Autodesk Inventor part; units mm, degrees
(part 2 of 2)
  line L285 (-19.9642, -36.6708) -> (-19.322, -36.6708)
  line L286 (-19.322, -36.6708) -> (-19.322, -35.0579)
  line L287 (-19.322, -35.0579) -> (-19.9642, -35.0579)
  line L288 (-19.9642, -35.0579) -> (-19.9642, -34.5614)
  spline S239 degree 2 poles (-19.9642, -34.5614) (-19.8234, -34.5614) (-19.5443, -34.5244) (-19.4603, -34.4848) knots 0 0 0 1 2 2 2
  spline S240 degree 2 poles (-19.4603, -34.4848) (-19.3639, -34.4354) (-19.2553, -34.27) (-19.2454, -34.1465) knots 0 0 0 1 2 2 2
  line L289 (-19.2454, -34.1465) -> (-18.5785, -34.1465)
  line L290 (-18.5785, -34.1465) -> (-18.5785, -36.6708)
  line L291 (-18.5785, -36.6708) -> (-17.9511, -36.6708)
  line L292 (-17.9511, -36.6708) -> (-17.9511, -37.2019)
  spline S241 degree 2 poles (-15.1624, -36.1645) (-15.1624, -36.6461) (-15.7725, -37.2661) (-16.3061, -37.2661) knots 0 0 0 1 2 2 2
  spline S242 degree 2 poles (-16.3061, -37.2661) (-16.5728, -37.2661) (-16.9903, -37.1129) (-17.136, -36.9623) knots 0 0 0 1 2 2 2
  spline S243 degree 2 poles (-17.136, -36.9623) (-17.3089, -36.7869) (-17.4941, -36.2312) (-17.4941, -35.8434) knots 0 0 0 1 2 2 2
  spline S244 degree 2 poles (-17.4941, -35.8434) (-17.4941, -35.4432) (-17.3212, -34.8208) (-17.1261, -34.5812) knots 0 0 0 1 2 2 2
  spline S245 degree 2 poles (-17.1261, -34.5812) (-16.9409, -34.3539) (-16.3382, -34.0971) (-15.9257, -34.0971) knots 0 0 0 1 2 2 2
  spline S246 degree 2 poles (-15.9257, -34.0971) (-15.775, -34.0971) (-15.4737, -34.1366) (-15.4193, -34.1489) knots 0 0 0 1 2 2 2
  line L293 (-15.4193, -34.1489) -> (-15.4193, -34.7467)
  line L294 (-15.4193, -34.7467) -> (-15.4737, -34.7467)
  spline S247 degree 2 poles (-15.4737, -34.7467) (-15.528, -34.7195) (-15.775, -34.6528) (-15.9331, -34.6528) knots 0 0 0 1 2 2 2
  spline S248 degree 2 poles (-15.9331, -34.6528) (-16.2912, -34.6528) (-16.6815, -35.0307) (-16.7284, -35.3815) knots 0 0 0 1 2 2 2
  spline S249 degree 2 poles (-16.7284, -35.3815) (-16.5778, -35.2851) (-16.269, -35.1715) (-16.0739, -35.1715) knots 0 0 0 1 2 2 2
  spline S250 degree 2 poles (-16.0739, -35.1715) (-15.9084, -35.1715) (-15.6194, -35.2604) (-15.5083, -35.3444) knots 0 0 0 1 2 2 2
  spline S251 degree 2 poles (-15.5083, -35.3444) (-15.3502, -35.4654) (-15.1624, -35.8582) (-15.1624, -36.1645) knots 0 0 0 1 2 2 2
  spline S252 degree 2 poles (-16.0541, -36.6239) (-15.9948, -36.5498) (-15.9306, -36.3769) (-15.9306, -36.2015) knots 0 0 0 1 2 2 2
  spline S253 degree 2 poles (-15.9306, -36.2015) (-15.9306, -36.0533) (-16.0047, -35.8606) (-16.0714, -35.8038) knots 0 0 0 1 2 2 2
  spline S254 degree 2 poles (-16.0714, -35.8038) (-16.1406, -35.7446) (-16.311, -35.7026) (-16.4073, -35.7026) knots 0 0 0 1 2 2 2
  spline S255 degree 2 poles (-16.4073, -35.7026) (-16.4888, -35.7026) (-16.6568, -35.7446) (-16.7309, -35.7742) knots 0 0 0 1 2 2 2
  spline S256 degree 2 poles (-16.7309, -35.7742) (-16.7309, -35.794) (-16.7359, -35.8878) (-16.7359, -35.9594) knots 0 0 0 1 2 2 2
  spline S257 degree 2 poles (-16.7359, -35.9594) (-16.7359, -36.2237) (-16.6445, -36.5424) (-16.5728, -36.6239) knots 0 0 0 1 2 2 2
  spline S258 degree 2 poles (-16.5728, -36.6239) (-16.521, -36.6906) (-16.3826, -36.7474) (-16.3085, -36.7474) knots 0 0 0 1 2 2 2
  spline S259 degree 2 poles (-16.3085, -36.7474) (-16.2468, -36.7474) (-16.1035, -36.6856) (-16.0541, -36.6239) knots 0 0 0 1 2 2 2
  line L295 (-12.8061, -37.2019) -> (-13.5224, -37.2019)
  line L296 (-13.5224, -37.2019) -> (-13.5224, -34.9023)
  line L297 (-13.5224, -34.9023) -> (-12.8061, -34.9023)
  line L298 (-12.8061, -34.9023) -> (-12.8061, -37.2019)
  line L299 (-12.7838, -34.5738) -> (-13.5421, -34.5738)
  line L300 (-13.5421, -34.5738) -> (-13.5421, -34.0155)
  line L301 (-13.5421, -34.0155) -> (-12.7838, -34.0155)
  line L302 (-12.7838, -34.0155) -> (-12.7838, -34.5738)
  line L303 (-10.1063, -37.2019) -> (-10.8276, -37.2019)
  line L304 (-10.8276, -37.2019) -> (-10.8276, -36.0632)
  spline S260 degree 2 poles (-10.8276, -36.0632) (-10.8276, -35.9224) (-10.8498, -35.6458) (-10.8794, -35.5815) knots 0 0 0 1 2 2 2
  spline S261 degree 2 poles (-10.8794, -35.5815) (-10.9165, -35.5025) (-11.0548, -35.4358) (-11.1734, -35.4358) knots 0 0 0 1 2 2 2
  spline S262 degree 2 poles (-11.1734, -35.4358) (-11.2598, -35.4358) (-11.4401, -35.5025) (-11.5414, -35.5741) knots 0 0 0 1 2 2 2
  line L305 (-11.5414, -35.5741) -> (-11.5414, -37.2019)
  line L306 (-11.5414, -37.2019) -> (-12.2577, -37.2019)
  line L307 (-12.2577, -37.2019) -> (-12.2577, -34.9023)
  line L308 (-12.2577, -34.9023) -> (-11.5414, -34.9023)
  line L309 (-11.5414, -34.9023) -> (-11.5414, -35.1567)
  spline S263 degree 2 poles (-11.5414, -35.1567) (-11.366, -35.0085) (-11.0326, -34.8405) (-10.83, -34.8405) knots 0 0 0 1 2 2 2
  spline S264 degree 2 poles (-10.83, -34.8405) (-10.4793, -34.8405) (-10.1063, -35.2851) (-10.1063, -35.705) knots 0 0 0 1 2 2 2
  line L310 (-10.1063, -35.705) -> (-10.1063, -37.2019)
  spline S265 degree 2 poles (-8.4489, -37.2636) (-8.733, -37.2636) (-9.2048, -37.1204) (-9.3801, -36.9722) knots 0 0 0 1 2 2 2
  spline S266 degree 2 poles (-9.3801, -36.9722) (-9.5506, -36.8215) (-9.7432, -36.3695) (-9.7432, -36.0632) knots 0 0 0 1 2 2 2
  spline S267 degree 2 poles (-9.7432, -36.0632) (-9.7432, -35.7322) (-9.5358, -35.2703) (-9.3554, -35.1221) knots 0 0 0 1 2 2 2
  spline S268 degree 2 poles (-9.3554, -35.1221) (-9.185, -34.9789) (-8.7206, -34.8405) (-8.4687, -34.8405) knots 0 0 0 1 2 2 2
  spline S269 degree 2 poles (-8.4687, -34.8405) (-8.2785, -34.8405) (-7.8981, -34.9295) (-7.7055, -35.0258) knots 0 0 0 1 2 2 2
  line L311 (-7.7055, -35.0258) -> (-7.7055, -35.6383)
  line L312 (-7.7055, -35.6383) -> (-7.7969, -35.6383)
  spline S270 degree 2 poles (-7.7969, -35.6383) (-7.8413, -35.5964) (-7.9648, -35.4976) (-8.0389, -35.458) knots 0 0 0 1 2 2 2
  spline S271 degree 2 poles (-8.0389, -35.458) (-8.118, -35.4136) (-8.3131, -35.3543) (-8.4341, -35.3543) knots 0 0 0 1 2 2 2
  spline S272 degree 2 poles (-8.4341, -35.3543) (-8.7083, -35.3543) (-9.0096, -35.7371) (-9.0096, -36.0632) knots 0 0 0 1 2 2 2
  spline S273 degree 2 poles (-9.0096, -36.0632) (-9.0096, -36.409) (-8.6885, -36.7499) (-8.4218, -36.7499) knots 0 0 0 1 2 2 2
  spline S274 degree 2 poles (-8.4218, -36.7499) (-8.2859, -36.7499) (-8.0834, -36.6881) (-8.0093, -36.6436) knots 0 0 0 1 2 2 2
  spline S275 degree 2 poles (-8.0093, -36.6436) (-7.9377, -36.6017) (-7.8339, -36.5078) (-7.7969, -36.4707) knots 0 0 0 1 2 2 2
  line L313 (-7.7969, -36.4707) -> (-7.7055, -36.4707)
  line L314 (-7.7055, -36.4707) -> (-7.7055, -37.0858)
  spline S276 degree 2 poles (-7.7055, -37.0858) (-7.7672, -37.1129) (-7.9278, -37.1821) (-8.0118, -37.2043) knots 0 0 0 1 2 2 2
  spline S277 degree 2 poles (-8.0118, -37.2043) (-8.1155, -37.234) (-8.2983, -37.2636) (-8.4489, -37.2636) knots 0 0 0 1 2 2 2
  line L315 (-5.2132, -37.2019) -> (-5.9345, -37.2019)
  line L316 (-5.9345, -37.2019) -> (-5.9345, -36.0632)
  spline S278 degree 2 poles (-5.9345, -36.0632) (-5.9345, -35.9224) (-5.9567, -35.6458) (-5.9863, -35.5815) knots 0 0 0 1 2 2 2
  spline S279 degree 2 poles (-5.9863, -35.5815) (-6.0234, -35.5025) (-6.1617, -35.4358) (-6.2803, -35.4358) knots 0 0 0 1 2 2 2
  spline S280 degree 2 poles (-6.2803, -35.4358) (-6.3667, -35.4358) (-6.547, -35.5025) (-6.6483, -35.5741) knots 0 0 0 1 2 2 2
  line L317 (-6.6483, -35.5741) -> (-6.6483, -37.2019)
  line L318 (-6.6483, -37.2019) -> (-7.3646, -37.2019)
  line L319 (-7.3646, -37.2019) -> (-7.3646, -34.018)
  line L320 (-7.3646, -34.018) -> (-6.6483, -34.018)
  line L321 (-6.6483, -34.018) -> (-6.6483, -35.1567)
  spline S281 degree 2 poles (-6.6483, -35.1567) (-6.4729, -35.0085) (-6.1395, -34.8405) (-5.9369, -34.8405) knots 0 0 0 1 2 2 2
  spline S282 degree 2 poles (-5.9369, -34.8405) (-5.5862, -34.8405) (-5.2132, -35.2851) (-5.2132, -35.705) knots 0 0 0 1 2 2 2
  line L322 (-5.2132, -35.705) -> (-5.2132, -37.2019)
  line L323 (7.0212, -34.759) -> (5.7195, -37.2019)
  line L324 (5.7195, -37.2019) -> (4.8698, -37.2019)
  line L325 (4.8698, -37.2019) -> (6.2307, -34.7294)
  line L326 (6.2307, -34.7294) -> (4.7784, -34.7294)
  line L327 (4.7784, -34.7294) -> (4.7784, -34.1539)
  line L328 (4.7784, -34.1539) -> (7.0212, -34.1539)
  line L329 (7.0212, -34.1539) -> (7.0212, -34.759)
  line L330 (9.2516, -34.018) -> (8.0388, -37.8638)
  line L331 (8.0388, -37.8638) -> (7.4509, -37.8638)
  line L332 (7.4509, -37.8638) -> (8.6612, -34.018)
  line L333 (8.6612, -34.018) -> (9.2516, -34.018)
  spline S283 degree 2 poles (12.1588, -36.1645) (12.1588, -36.6461) (11.5487, -37.2661) (11.0152, -37.2661) knots 0 0 0 1 2 2 2
  spline S284 degree 2 poles (11.0152, -37.2661) (10.7484, -37.2661) (10.331, -37.1129) (10.1852, -36.9623) knots 0 0 0 1 2 2 2
  spline S285 degree 2 poles (10.1852, -36.9623) (10.0123, -36.7869) (9.8271, -36.2312) (9.8271, -35.8434) knots 0 0 0 1 2 2 2
  spline S286 degree 2 poles (9.8271, -35.8434) (9.8271, -35.4432) (10, -34.8208) (10.1951, -34.5812) knots 0 0 0 1 2 2 2
  spline S287 degree 2 poles (10.1951, -34.5812) (10.3804, -34.3539) (10.9831, -34.0971) (11.3956, -34.0971) knots 0 0 0 1 2 2 2
  spline S288 degree 2 poles (11.3956, -34.0971) (11.5462, -34.0971) (11.8476, -34.1366) (11.9019, -34.1489) knots 0 0 0 1 2 2 2
  line L334 (11.9019, -34.1489) -> (11.9019, -34.7467)
  line L335 (11.9019, -34.7467) -> (11.8476, -34.7467)
  spline S289 degree 2 poles (11.8476, -34.7467) (11.7932, -34.7195) (11.5462, -34.6528) (11.3881, -34.6528) knots 0 0 0 1 2 2 2
  spline S290 degree 2 poles (11.3881, -34.6528) (11.03, -34.6528) (10.6397, -35.0307) (10.5928, -35.3815) knots 0 0 0 1 2 2 2
  spline S291 degree 2 poles (10.5928, -35.3815) (10.7435, -35.2851) (11.0522, -35.1715) (11.2474, -35.1715) knots 0 0 0 1 2 2 2
  spline S292 degree 2 poles (11.2474, -35.1715) (11.4128, -35.1715) (11.7018, -35.2604) (11.813, -35.3444) knots 0 0 0 1 2 2 2
  spline S293 degree 2 poles (11.813, -35.3444) (11.9711, -35.4654) (12.1588, -35.8582) (12.1588, -36.1645) knots 0 0 0 1 2 2 2
  spline S294 degree 2 poles (11.2671, -36.6239) (11.3264, -36.5498) (11.3906, -36.3769) (11.3906, -36.2015) knots 0 0 0 1 2 2 2
  spline S295 degree 2 poles (11.3906, -36.2015) (11.3906, -36.0533) (11.3165, -35.8606) (11.2498, -35.8038) knots 0 0 0 1 2 2 2
  spline S296 degree 2 poles (11.2498, -35.8038) (11.1807, -35.7446) (11.0102, -35.7026) (10.9139, -35.7026) knots 0 0 0 1 2 2 2
  spline S297 degree 2 poles (10.9139, -35.7026) (10.8324, -35.7026) (10.6644, -35.7446) (10.5903, -35.7742) knots 0 0 0 1 2 2 2
  spline S298 degree 2 poles (10.5903, -35.7742) (10.5903, -35.794) (10.5854, -35.8878) (10.5854, -35.9594) knots 0 0 0 1 2 2 2
  spline S299 degree 2 poles (10.5854, -35.9594) (10.5854, -36.2237) (10.6768, -36.5424) (10.7484, -36.6239) knots 0 0 0 1 2 2 2
  spline S300 degree 2 poles (10.7484, -36.6239) (10.8003, -36.6906) (10.9386, -36.7474) (11.0127, -36.7474) knots 0 0 0 1 2 2 2
  spline S301 degree 2 poles (11.0127, -36.7474) (11.0744, -36.7474) (11.2177, -36.6856) (11.2671, -36.6239) knots 0 0 0 1 2 2 2
  line L336 (14.5152, -37.2019) -> (13.7989, -37.2019)
  line L337 (13.7989, -37.2019) -> (13.7989, -34.9023)
  line L338 (13.7989, -34.9023) -> (14.5152, -34.9023)
  line L339 (14.5152, -34.9023) -> (14.5152, -37.2019)
  line L340 (14.5374, -34.5738) -> (13.7791, -34.5738)
  line L341 (13.7791, -34.5738) -> (13.7791, -34.0155)
  line L342 (13.7791, -34.0155) -> (14.5374, -34.0155)
  line L343 (14.5374, -34.0155) -> (14.5374, -34.5738)
  line L344 (17.2149, -37.2019) -> (16.4937, -37.2019)
  line L345 (16.4937, -37.2019) -> (16.4937, -36.0632)
  spline S302 degree 2 poles (16.4937, -36.0632) (16.4937, -35.9224) (16.4714, -35.6458) (16.4418, -35.5815) knots 0 0 0 1 2 2 2
  spline S303 degree 2 poles (16.4418, -35.5815) (16.4047, -35.5025) (16.2664, -35.4358) (16.1479, -35.4358) knots 0 0 0 1 2 2 2
  spline S304 degree 2 poles (16.1479, -35.4358) (16.0614, -35.4358) (15.8811, -35.5025) (15.7798, -35.5741) knots 0 0 0 1 2 2 2
  line L346 (15.7798, -35.5741) -> (15.7798, -37.2019)
  line L347 (15.7798, -37.2019) -> (15.0635, -37.2019)
  line L348 (15.0635, -37.2019) -> (15.0635, -34.9023)
  line L349 (15.0635, -34.9023) -> (15.7798, -34.9023)
  line L350 (15.7798, -34.9023) -> (15.7798, -35.1567)
  spline S305 degree 2 poles (15.7798, -35.1567) (15.9552, -35.0085) (16.2887, -34.8405) (16.4912, -34.8405) knots 0 0 0 1 2 2 2
  spline S306 degree 2 poles (16.4912, -34.8405) (16.8419, -34.8405) (17.2149, -35.2851) (17.2149, -35.705) knots 0 0 0 1 2 2 2
  line L351 (17.2149, -35.705) -> (17.2149, -37.2019)
  spline S307 degree 2 poles (18.8723, -37.2636) (18.5882, -37.2636) (18.1165, -37.1204) (17.9411, -36.9722) knots 0 0 0 1 2 2 2
  spline S308 degree 2 poles (17.9411, -36.9722) (17.7707, -36.8215) (17.578, -36.3695) (17.578, -36.0632) knots 0 0 0 1 2 2 2
  spline S309 degree 2 poles (17.578, -36.0632) (17.578, -35.7322) (17.7855, -35.2703) (17.9658, -35.1221) knots 0 0 0 1 2 2 2
  spline S310 degree 2 poles (17.9658, -35.1221) (18.1362, -34.9789) (18.6006, -34.8405) (18.8525, -34.8405) knots 0 0 0 1 2 2 2
  spline S311 degree 2 poles (18.8525, -34.8405) (19.0427, -34.8405) (19.4231, -34.9295) (19.6158, -35.0258) knots 0 0 0 1 2 2 2
  line L352 (19.6158, -35.0258) -> (19.6158, -35.6383)
  line L353 (19.6158, -35.6383) -> (19.5244, -35.6383)
  spline S312 degree 2 poles (19.5244, -35.6383) (19.4799, -35.5964) (19.3564, -35.4976) (19.2823, -35.458) knots 0 0 0 1 2 2 2
  spline S313 degree 2 poles (19.2823, -35.458) (19.2033, -35.4136) (19.0081, -35.3543) (18.8871, -35.3543) knots 0 0 0 1 2 2 2
  spline S314 degree 2 poles (18.8871, -35.3543) (18.6129, -35.3543) (18.3116, -35.7371) (18.3116, -36.0632) knots 0 0 0 1 2 2 2
  spline S315 degree 2 poles (18.3116, -36.0632) (18.3116, -36.409) (18.6327, -36.7499) (18.8995, -36.7499) knots 0 0 0 1 2 2 2
  spline S316 degree 2 poles (18.8995, -36.7499) (19.0353, -36.7499) (19.2379, -36.6881) (19.312, -36.6436) knots 0 0 0 1 2 2 2
  spline S317 degree 2 poles (19.312, -36.6436) (19.3836, -36.6017) (19.4873, -36.5078) (19.5244, -36.4707) knots 0 0 0 1 2 2 2
  line L354 (19.5244, -36.4707) -> (19.6158, -36.4707)
  line L355 (19.6158, -36.4707) -> (19.6158, -37.0858)
  spline S318 degree 2 poles (19.6158, -37.0858) (19.554, -37.1129) (19.3935, -37.1821) (19.3095, -37.2043) knots 0 0 0 1 2 2 2
  spline S319 degree 2 poles (19.3095, -37.2043) (19.2057, -37.234) (19.023, -37.2636) (18.8723, -37.2636) knots 0 0 0 1 2 2 2
  line L356 (22.108, -37.2019) -> (21.3868, -37.2019)
  line L357 (21.3868, -37.2019) -> (21.3868, -36.0632)
  spline S320 degree 2 poles (21.3868, -36.0632) (21.3868, -35.9224) (21.3645, -35.6458) (21.3349, -35.5815) knots 0 0 0 1 2 2 2
  spline S321 degree 2 poles (21.3349, -35.5815) (21.2978, -35.5025) (21.1595, -35.4358) (21.041, -35.4358) knots 0 0 0 1 2 2 2
  spline S322 degree 2 poles (21.041, -35.4358) (20.9545, -35.4358) (20.7742, -35.5025) (20.6729, -35.5741) knots 0 0 0 1 2 2 2
  line L358 (20.6729, -35.5741) -> (20.6729, -37.2019)
  line L359 (20.6729, -37.2019) -> (19.9566, -37.2019)
  line L360 (19.9566, -37.2019) -> (19.9566, -34.018)
  line L361 (19.9566, -34.018) -> (20.6729, -34.018)
  line L362 (20.6729, -34.018) -> (20.6729, -35.1567)
  spline S323 degree 2 poles (20.6729, -35.1567) (20.8483, -35.0085) (21.1818, -34.8405) (21.3843, -34.8405) knots 0 0 0 1 2 2 2
  spline S324 degree 2 poles (21.3843, -34.8405) (21.735, -34.8405) (22.108, -35.2851) (22.108, -35.705) knots 0 0 0 1 2 2 2
  line L363 (22.108, -35.705) -> (22.108, -37.2019)
  spline S325 degree 2 poles (37.5726, -36.2781) (37.5726, -36.5029) (37.4071, -36.8709) (37.2465, -36.9993) knots 0 0 0 1 2 2 2
  spline S326 degree 2 poles (37.2465, -36.9993) (37.086, -37.1278) (36.6488, -37.2661) (36.3351, -37.2661) knots 0 0 0 1 2 2 2
  spline S327 degree 2 poles (36.3351, -37.2661) (35.9794, -37.2661) (35.4706, -37.1475) (35.31, -37.0734) knots 0 0 0 1 2 2 2
  line L364 (35.31, -37.0734) -> (35.31, -36.4115)
  line L365 (35.31, -36.4115) -> (35.3841, -36.4115)
  spline S328 degree 2 poles (35.3841, -36.4115) (35.5521, -36.5177) (36.0041, -36.6758) (36.1918, -36.6758) knots 0 0 0 1 2 2 2
  spline S329 degree 2 poles (36.1918, -36.6758) (36.303, -36.6758) (36.5623, -36.6362) (36.6512, -36.572) knots 0 0 0 1 2 2 2
  spline S330 degree 2 poles (36.6512, -36.572) (36.7204, -36.5201) (36.8044, -36.3695) (36.8044, -36.2336) knots 0 0 0 1 2 2 2
  spline S331 degree 2 poles (36.8044, -36.2336) (36.8044, -36.0978) (36.6858, -35.952) (36.587, -35.9175) knots 0 0 0 1 2 2 2
  spline S332 degree 2 poles (36.587, -35.9175) (36.4882, -35.8829) (36.214, -35.8755) (36.1078, -35.8755) knots 0 0 0 1 2 2 2
  line L366 (36.1078, -35.8755) -> (35.9769, -35.8755)
  line L367 (35.9769, -35.8755) -> (35.9769, -35.3395)
  line L368 (35.9769, -35.3395) -> (36.098, -35.3395)
  spline S333 degree 2 poles (36.098, -35.3395) (36.2363, -35.3395) (36.4709, -35.3148) (36.5524, -35.2777) knots 0 0 0 1 2 2 2
  spline S334 degree 2 poles (36.5524, -35.2777) (36.6339, -35.2382) (36.7253, -35.0999) (36.7253, -34.9813) knots 0 0 0 1 2 2 2
  spline S335 degree 2 poles (36.7253, -34.9813) (36.7253, -34.8875) (36.6389, -34.7714) (36.5771, -34.7393) knots 0 0 0 1 2 2 2
  spline S336 degree 2 poles (36.5771, -34.7393) (36.503, -34.7022) (36.3054, -34.6775) (36.2363, -34.6775) knots 0 0 0 1 2 2 2
  spline S337 degree 2 poles (36.2363, -34.6775) (36.1251, -34.6775) (35.8905, -34.7294) (35.7818, -34.7714) knots 0 0 0 1 2 2 2
  spline S338 degree 2 poles (35.7818, -34.7714) (35.6953, -34.8035) (35.5076, -34.9072) (35.4632, -34.9344) knots 0 0 0 1 2 2 2
  line L369 (35.4632, -34.9344) -> (35.3989, -34.9344)
  line L370 (35.3989, -34.9344) -> (35.3989, -34.2823)
  spline S339 degree 2 poles (35.3989, -34.2823) (35.557, -34.2156) (36.0905, -34.0896) (36.3697, -34.0896) knots 0 0 0 1 2 2 2
  spline S340 degree 2 poles (36.3697, -34.0896) (36.6414, -34.0896) (37.0415, -34.1835) (37.1823, -34.2749) knots 0 0 0 1 2 2 2
  spline S341 degree 2 poles (37.1823, -34.2749) (37.3379, -34.3712) (37.4935, -34.6676) (37.4935, -34.8529) knots 0 0 0 1 2 2 2
  spline S342 degree 2 poles (37.4935, -34.8529) (37.4935, -35.1147) (37.1922, -35.505) (36.9452, -35.5618) knots 0 0 0 1 2 2 2
  line L371 (36.9452, -35.5618) -> (36.9452, -35.5914)
  spline S343 degree 2 poles (36.9452, -35.5914) (37.0538, -35.6062) (37.2613, -35.6853) (37.3601, -35.7742) knots 0 0 0 1 2 2 2
  spline S344 degree 2 poles (37.3601, -35.7742) (37.4515, -35.8532) (37.5726, -36.1052) (37.5726, -36.2781) knots 0 0 0 1 2 2 2
  line L372 (39.8129, -34.018) -> (38.6001, -37.8638)
  line L373 (38.6001, -37.8638) -> (38.0122, -37.8638)
  line L374 (38.0122, -37.8638) -> (39.2225, -34.018)
  line L375 (39.2225, -34.018) -> (39.8129, -34.018)
  spline S345 degree 2 poles (42.7299, -36.3547) (42.7299, -36.5498) (42.5669, -36.8882) (42.4113, -37.0117) knots 0 0 0 1 2 2 2
  spline S346 degree 2 poles (42.4113, -37.0117) (42.2557, -37.1352) (41.8086, -37.2735) (41.5196, -37.2735) knots 0 0 0 1 2 2 2
  spline S347 degree 2 poles (41.5196, -37.2735) (41.2109, -37.2735) (40.749, -37.1327) (40.6008, -37.0117) knots 0 0 0 1 2 2 2
  spline S348 degree 2 poles (40.6008, -37.0117) (40.4551, -36.8906) (40.3167, -36.5621) (40.3167, -36.3794) knots 0 0 0 1 2 2 2
  spline S349 degree 2 poles (40.3167, -36.3794) (40.3167, -36.1175) (40.6057, -35.7693) (40.8799, -35.6532) knots 0 0 0 1 2 2 2
  line L376 (40.8799, -35.6532) -> (40.8799, -35.6408)
  spline S350 degree 2 poles (40.8799, -35.6408) (40.6107, -35.5099) (40.3983, -35.1369) (40.3983, -34.9072) knots 0 0 0 1 2 2 2
  spline S351 degree 2 poles (40.3983, -34.9072) (40.3983, -34.7393) (40.5465, -34.4453) (40.6922, -34.3292) knots 0 0 0 1 2 2 2
  spline S352 degree 2 poles (40.6922, -34.3292) (40.833, -34.2181) (41.2603, -34.0847) (41.527, -34.0847) knots 0 0 0 1 2 2 2
  spline S353 degree 2 poles (41.527, -34.0847) (41.8086, -34.0847) (42.2285, -34.2057) (42.3644, -34.3045) knots 0 0 0 1 2 2 2
  spline S354 degree 2 poles (42.3644, -34.3045) (42.5027, -34.4033) (42.6509, -34.6899) (42.6509, -34.8554) knots 0 0 0 1 2 2 2
  spline S355 degree 2 poles (42.6509, -34.8554) (42.6509, -35.0727) (42.399, -35.421) (42.1396, -35.542) knots 0 0 0 1 2 2 2
  line L377 (42.1396, -35.542) -> (42.1396, -35.5519)
  spline S356 degree 2 poles (42.1396, -35.5519) (42.4434, -35.6754) (42.7299, -36.0755) (42.7299, -36.3547) knots 0 0 0 1 2 2 2
  spline S357 degree 2 poles (41.9741, -36.3868) (41.9741, -36.2361) (41.8457, -36.078) (41.6382, -35.9767) knots 0 0 0 1 2 2 2
  spline S358 degree 2 poles (41.6382, -35.9767) (41.5789, -35.9496) (41.3541, -35.8631) (41.2677, -35.8261) knots 0 0 0 1 2 2 2
  spline S359 degree 2 poles (41.2677, -35.8261) (41.1887, -35.9051) (41.0627, -36.1422) (41.0627, -36.283) knots 0 0 0 1 2 2 2
  spline S360 degree 2 poles (41.0627, -36.283) (41.0627, -36.4954) (41.3344, -36.7499) (41.5542, -36.7499) knots 0 0 0 1 2 2 2
  spline S361 degree 2 poles (41.5542, -36.7499) (41.616, -36.7499) (41.7691, -36.7103) (41.8284, -36.6708) knots 0 0 0 1 2 2 2
  spline S362 degree 2 poles (41.8284, -36.6708) (41.8951, -36.6239) (41.9741, -36.4954) (41.9741, -36.3868) knots 0 0 0 1 2 2 2
  spline S363 degree 2 poles (41.9074, -34.9443) (41.9074, -34.7887) (41.7024, -34.6034) (41.527, -34.6034) knots 0 0 0 1 2 2 2
  spline S364 degree 2 poles (41.527, -34.6034) (41.3591, -34.6034) (41.1541, -34.7714) (41.1541, -34.8949) knots 0 0 0 1 2 2 2
  spline S365 degree 2 poles (41.1541, -34.8949) (41.1541, -35.0159) (41.2776, -35.1666) (41.4085, -35.2283) knots 0 0 0 1 2 2 2
  spline S366 degree 2 poles (41.4085, -35.2283) (41.4653, -35.258) (41.6234, -35.3197) (41.7543, -35.3691) knots 0 0 0 1 2 2 2
  spline S367 degree 2 poles (41.7543, -35.3691) (41.8333, -35.2654) (41.9074, -35.0702) (41.9074, -34.9443) knots 0 0 0 1 2 2 2
  line L378 (45.0765, -37.2019) -> (44.3602, -37.2019)
  line L379 (44.3602, -37.2019) -> (44.3602, -34.9023)
  line L380 (44.3602, -34.9023) -> (45.0765, -34.9023)
  line L381 (45.0765, -34.9023) -> (45.0765, -37.2019)
  line L382 (45.0987, -34.5738) -> (44.3404, -34.5738)
  line L383 (44.3404, -34.5738) -> (44.3404, -34.0155)
  line L384 (44.3404, -34.0155) -> (45.0987, -34.0155)
  line L385 (45.0987, -34.0155) -> (45.0987, -34.5738)
  line L386 (47.7762, -37.2019) -> (47.0549, -37.2019)
  line L387 (47.0549, -37.2019) -> (47.0549, -36.0632)
  spline S368 degree 2 poles (47.0549, -36.0632) (47.0549, -35.9224) (47.0327, -35.6458) (47.0031, -35.5815) knots 0 0 0 1 2 2 2
  spline S369 degree 2 poles (47.0031, -35.5815) (46.966, -35.5025) (46.8277, -35.4358) (46.7091, -35.4358) knots 0 0 0 1 2 2 2
  spline S370 degree 2 poles (46.7091, -35.4358) (46.6227, -35.4358) (46.4424, -35.5025) (46.3411, -35.5741) knots 0 0 0 1 2 2 2
  line L388 (46.3411, -35.5741) -> (46.3411, -37.2019)
  line L389 (46.3411, -37.2019) -> (45.6248, -37.2019)
  line L390 (45.6248, -37.2019) -> (45.6248, -34.9023)
  line L391 (45.6248, -34.9023) -> (46.3411, -34.9023)
  line L392 (46.3411, -34.9023) -> (46.3411, -35.1567)
  spline S371 degree 2 poles (46.3411, -35.1567) (46.5165, -35.0085) (46.8499, -34.8405) (47.0525, -34.8405) knots 0 0 0 1 2 2 2
  spline S372 degree 2 poles (47.0525, -34.8405) (47.4032, -34.8405) (47.7762, -35.2851) (47.7762, -35.705) knots 0 0 0 1 2 2 2
  line L393 (47.7762, -35.705) -> (47.7762, -37.2019)
  spline S373 degree 2 poles (49.4336, -37.2636) (49.1495, -37.2636) (48.6777, -37.1204) (48.5024, -36.9722) knots 0 0 0 1 2 2 2
  spline S374 degree 2 poles (48.5024, -36.9722) (48.3319, -36.8215) (48.1393, -36.3695) (48.1393, -36.0632) knots 0 0 0 1 2 2 2
  spline S375 degree 2 poles (48.1393, -36.0632) (48.1393, -35.7322) (48.3468, -35.2703) (48.5271, -35.1221) knots 0 0 0 1 2 2 2
  spline S376 degree 2 poles (48.5271, -35.1221) (48.6975, -34.9789) (49.1619, -34.8405) (49.4138, -34.8405) knots 0 0 0 1 2 2 2
  spline S377 degree 2 poles (49.4138, -34.8405) (49.604, -34.8405) (49.9844, -34.9295) (50.177, -35.0258) knots 0 0 0 1 2 2 2
  line L394 (50.177, -35.0258) -> (50.177, -35.6383)
  line L395 (50.177, -35.6383) -> (50.0857, -35.6383)
  spline S378 degree 2 poles (50.0857, -35.6383) (50.0412, -35.5964) (49.9177, -35.4976) (49.8436, -35.458) knots 0 0 0 1 2 2 2
  spline S379 degree 2 poles (49.8436, -35.458) (49.7646, -35.4136) (49.5694, -35.3543) (49.4484, -35.3543) knots 0 0 0 1 2 2 2
  spline S380 degree 2 poles (49.4484, -35.3543) (49.1742, -35.3543) (48.8729, -35.7371) (48.8729, -36.0632) knots 0 0 0 1 2 2 2
  spline S381 degree 2 poles (48.8729, -36.0632) (48.8729, -36.409) (49.194, -36.7499) (49.4607, -36.7499) knots 0 0 0 1 2 2 2
  spline S382 degree 2 poles (49.4607, -36.7499) (49.5966, -36.7499) (49.7991, -36.6881) (49.8732, -36.6436) knots 0 0 0 1 2 2 2
  spline S383 degree 2 poles (49.8732, -36.6436) (49.9449, -36.6017) (50.0486, -36.5078) (50.0857, -36.4707) knots 0 0 0 1 2 2 2
  line L396 (50.0857, -36.4707) -> (50.177, -36.4707)
  line L397 (50.177, -36.4707) -> (50.177, -37.0858)
  spline S384 degree 2 poles (50.177, -37.0858) (50.1153, -37.1129) (49.9547, -37.1821) (49.8708, -37.2043) knots 0 0 0 1 2 2 2
  spline S385 degree 2 poles (49.8708, -37.2043) (49.767, -37.234) (49.5842, -37.2636) (49.4336, -37.2636) knots 0 0 0 1 2 2 2
  line L398 (52.6693, -37.2019) -> (51.948, -37.2019)
  line L399 (51.948, -37.2019) -> (51.948, -36.0632)
  spline S386 degree 2 poles (51.948, -36.0632) (51.948, -35.9224) (51.9258, -35.6458) (51.8962, -35.5815) knots 0 0 0 1 2 2 2
  spline S387 degree 2 poles (51.8962, -35.5815) (51.8591, -35.5025) (51.7208, -35.4358) (51.6022, -35.4358) knots 0 0 0 1 2 2 2
  spline S388 degree 2 poles (51.6022, -35.4358) (51.5158, -35.4358) (51.3355, -35.5025) (51.2342, -35.5741) knots 0 0 0 1 2 2 2
  line L400 (51.2342, -35.5741) -> (51.2342, -37.2019)
  line L401 (51.2342, -37.2019) -> (50.5179, -37.2019)
  line L402 (50.5179, -37.2019) -> (50.5179, -34.018)
  line L403 (50.5179, -34.018) -> (51.2342, -34.018)
  line L404 (51.2342, -34.018) -> (51.2342, -35.1567)
  spline S389 degree 2 poles (51.2342, -35.1567) (51.4096, -35.0085) (51.743, -34.8405) (51.9456, -34.8405) knots 0 0 0 1 2 2 2
  spline S390 degree 2 poles (51.9456, -34.8405) (52.2963, -34.8405) (52.6693, -35.2851) (52.6693, -35.705) knots 0 0 0 1 2 2 2
  line L405 (52.6693, -35.705) -> (52.6693, -37.2019)
  point P0 (0, 0)
  dimension "d45" = 8.7721
  dimension "d46" = 40.64
  dimension "d50" = 90
  dimension "d52" = 90
  dimension "d53" = 90
  dimension "d54" = 90
  dimension "d55" = 90
  dimension "d56" = 90
  constraints: 48 end point, 15 horizontal, 14 point on circle, 7 parallel, 3 collinear, 3 tangent, 2 perpendicular, 2 vertical, 1 horizontal alignment, 1 other
  measures "d45" distance between parallel lines of L1 L0
  measures "d46" distance between parallel lines of L5 L0
  measures "d50" angle of L9 L2
  measures "d52" angle of L11 L1
  measures "d53" angle of L13 L3
  measures "d54" angle of L15 L4
  measures "d55" angle of L19 L6
  measures "d56" angle of L21 L7
extrude "textLabels" cut sketch "Sketch7" against normal blind 3.175
fillet "Fillet1" radius 3.175 8 edges at (-53.7972, 0, -12.7) (-27.8384, 0, -12.7) (1.9304, 0, -12.7) (31.4452, 0, -12.7) (36.6471, 0, 19.05) (6.9748, 0, 19.05) (-20.6654, 0, 19.05) (-46.7817, 0, 19.05)
fillet "Fillet2" radius 3.175 4 edges at (-63.5, -3.175, 44.45) (-63.5, -3.175, -44.45) (63.5, -3.175, 44.45) (63.5, -3.175, -44.45)
equation "\"gap0\" = frontGapBetweenHoles"
equation "\"gap1\" = 0.5 * hex5_16inchHole + 0.5 * hex1_4inchHole + frontGapBetweenHoles"
equation "\"gap2\" = 0.5 * hex3_8inchHole + 0.5 * hex5_16inchHole + frontGapBetweenHoles"
equation "\"gap3\" = 0.5 * hex7_16inchHole + 0.5 * hex3_8inchHole + frontGapBetweenHoles"
equation "\"gap5\" = backGapBetweenHoles"
equation "\"gap6\" = 0.5 * hex9_16inchHole + 0.5 * hex1_2inchHole + backGapBetweenHoles"
equation "\"gap7\" = 0.5 * hex5_8inchHole + 0.5 * hex9_16inchHole + backGapBetweenHoles"
equation "\"gap8\" = 0.5 * hex3_4inchHole + 0.5 * hex5_8inchHole + backGapBetweenHoles"
equation "\"d46\" = centerLineForBackText"
equation "\"frontGapBetweenHoles\" = 16.71828"
equation "\"backGapBetweenHoles\" = 9.7028"
equation "\"centerLineForFrontText\" = 8.3185"
equation "\"centerLineForBackText\" = 40.64"
body "Solid1"
